Autodesk Inventor part; units mm, degrees
(part 2 of 2)
  spline S30 degree 3 poles (-13.3433, 65.0371) (-13.2374, 65.0737) (-13.0255, 65.1467) (-12.7024, 65.2399) (-12.4302, 65.3065) (-12.2106, 65.3513) (-12.0451, 65.3806) (-11.8787, 65.4045) (-11.6563, 65.4323) (-11.4592, 65.431) (-11.2933, 65.4596) (-11.2263, 65.4806) (-11.175, 65.5032) (-11.1385, 65.5242) (-11.1036, 65.5476) (-11.0712, 65.5745) (-11.0418, 65.6046) (-11.0157, 65.6376) (-10.9923, 65.6726) (-10.9749, 65.7109) (-10.9587, 65.7498) (-10.9463, 65.8046) (-10.9343, 65.8736) (-10.92, 65.9421) (-10.9113, 65.9976) (-10.912, 66.0397) (-10.914, 66.0817) (-10.9229, 66.1229) (-10.9349, 66.1632) (-10.9512, 66.202) (-10.9713, 66.239) (-10.9951, 66.2736) (-11.0213, 66.3066) (-11.0607, 66.3465) (-11.1152, 66.3908) (-11.2588, 66.4786) (-11.4424, 66.5501) (-11.6389, 66.658) (-11.7847, 66.7417) (-11.9277, 66.83) (-12.1153, 66.9527) (-12.3437, 67.115) (-12.6096, 67.3209) (-12.7795, 67.467) (-12.8645, 67.5401) knots 0 0 0 0 0.033613 0.067227 0.100839 0.117647 0.134454 0.151261 0.168068 0.201677 0.210077 0.218473 0.222676 0.226878 0.231076 0.235279 0.239479 0.24368 0.247882 0.252083 0.256283 0.260485 0.268889 0.277292 0.281494 0.285694 0.289895 0.294097 0.298298 0.302498 0.306701 0.310899 0.315101 0.319304 0.3277 0.3361 0.369709 0.386516 0.403323 0.420131 0.436938 0.470551 0.504164 0.537777 0.537777 0.537777 0.537777 projected
  arc A30 (-13.3433, 65.0371) -> (-13.4236, 64.2845) centre (6.5, 62.5385) ccw projected
  spline S31 degree 3 poles (-13.4839, 61.7369) (-13.3855, 61.7904) (-13.1885, 61.8974) (-12.8852, 62.0425) (-12.6276, 62.1529) (-12.4184, 62.2332) (-12.26, 62.2894) (-12.0998, 62.3404) (-11.885, 62.4044) (-11.6904, 62.4355) (-11.5315, 62.4911) (-11.4688, 62.5229) (-11.4219, 62.5536) (-11.3894, 62.5803) (-11.3588, 62.6091) (-11.3313, 62.641) (-11.3072, 62.6755) (-11.2869, 62.7123) (-11.2696, 62.7507) (-11.2587, 62.7914) (-11.2491, 62.8324) (-11.246, 62.8885) (-11.2455, 62.9585) (-11.2427, 63.0284) (-11.2432, 63.0846) (-11.2508, 63.126) (-11.2597, 63.1671) (-11.2752, 63.2063) (-11.2937, 63.2441) (-11.3162, 63.2797) (-11.3421, 63.3128) (-11.3713, 63.3431) (-11.4025, 63.3713) (-11.448, 63.4042) (-11.509, 63.4389) (-11.6652, 63.5019) (-11.858, 63.5422) (-12.0696, 63.6163) (-12.2272, 63.6748) (-12.3828, 63.7384) (-12.588, 63.8285) (-12.84, 63.951) (-13.1361, 64.1103) (-13.3278, 64.2265) (-13.4236, 64.2845) knots 0 0 0 0 0.033613 0.067227 0.100839 0.117647 0.134454 0.151261 0.168068 0.201677 0.210077 0.218473 0.222676 0.226878 0.231076 0.235279 0.239479 0.24368 0.247882 0.252083 0.256283 0.260485 0.268889 0.277292 0.281494 0.285694 0.289895 0.294097 0.298298 0.302498 0.306701 0.310899 0.315101 0.319304 0.3277 0.3361 0.369709 0.386516 0.403323 0.420131 0.436938 0.470551 0.504164 0.537777 0.537777 0.537777 0.537777 projected
  arc A31 (-13.4839, 61.7369) -> (-13.4393, 60.9814) centre (6.5, 62.5385) ccw projected
  spline S32 degree 3 poles (-13.0795, 58.4586) (-12.9911, 58.5276) (-12.8145, 58.6655) (-12.5391, 58.8586) (-12.3033, 59.0099) (-12.1101, 59.1235) (-11.9631, 59.205) (-11.8135, 59.2817) (-11.6121, 59.3802) (-11.4254, 59.4429) (-11.2777, 59.5238) (-11.2212, 59.5655) (-11.1799, 59.6035) (-11.1523, 59.6352) (-11.1268, 59.6687) (-11.105, 59.7046) (-11.0869, 59.7426) (-11.0729, 59.7823) (-11.0621, 59.8231) (-11.0581, 59.865) (-11.0554, 59.907) (-11.0616, 59.9628) (-11.0726, 60.0319) (-11.0813, 60.1014) (-11.0911, 60.1567) (-11.1054, 60.1963) (-11.121, 60.2354) (-11.1427, 60.2715) (-11.1672, 60.3057) (-11.1952, 60.3371) (-11.2262, 60.3655) (-11.26, 60.3906) (-11.2954, 60.4133) (-11.3457, 60.4382) (-11.4116, 60.4624) (-11.576, 60.4989) (-11.7728, 60.5068) (-11.9937, 60.5451) (-12.1588, 60.5769) (-12.3227, 60.614) (-12.54, 60.6692) (-12.8087, 60.7485) (-13.127, 60.8569) (-13.3352, 60.9399) (-13.4393, 60.9814) knots 0 0 0 0 0.033613 0.067227 0.100839 0.117647 0.134454 0.151261 0.168068 0.201677 0.210077 0.218473 0.222676 0.226878 0.231076 0.235279 0.239479 0.24368 0.247882 0.252083 0.256283 0.260485 0.268889 0.277292 0.281494 0.285694 0.289895 0.294097 0.298298 0.302498 0.306701 0.310899 0.315101 0.319304 0.3277 0.3361 0.369709 0.386516 0.403323 0.420131 0.436938 0.470551 0.504164 0.537777 0.537777 0.537777 0.537777 projected
  arc A32 (-13.0795, 58.4586) -> (-12.9111, 57.7207) centre (6.5, 62.5385) ccw projected
  spline S33 degree 3 poles (-12.1409, 55.2916) (-12.0651, 55.3741) (-11.9136, 55.5393) (-11.6738, 55.775) (-11.466, 55.9631) (-11.2942, 56.107) (-11.1626, 56.2116) (-11.0277, 56.3118) (-10.8453, 56.4421) (-10.6714, 56.5347) (-10.5391, 56.6388) (-10.4902, 56.6892) (-10.4557, 56.7335) (-10.4337, 56.7693) (-10.4141, 56.8065) (-10.3984, 56.8456) (-10.3869, 56.8861) (-10.3796, 56.9275) (-10.3757, 56.9695) (-10.3786, 57.0114) (-10.3829, 57.0533) (-10.3981, 57.1074) (-10.4204, 57.1738) (-10.4404, 57.2408) (-10.4591, 57.2938) (-10.4798, 57.3305) (-10.5016, 57.3665) (-10.529, 57.3985) (-10.5587, 57.4282) (-10.5915, 57.4546) (-10.6268, 57.4775) (-10.6643, 57.4967) (-10.7029, 57.5132) (-10.7566, 57.5296) (-10.8256, 57.5426) (-10.9937, 57.5515) (-11.1892, 57.5269) (-11.4134, 57.5283) (-11.5814, 57.5325) (-11.7493, 57.5422) (-11.9726, 57.5608) (-12.2507, 57.5948) (-12.5826, 57.6493) (-12.8016, 57.6969) (-12.9111, 57.7207) knots 0 0 0 0 0.033613 0.067227 0.100839 0.117647 0.134454 0.151261 0.168068 0.201677 0.210077 0.218473 0.222676 0.226878 0.231076 0.235279 0.239479 0.24368 0.247882 0.252083 0.256283 0.260485 0.268889 0.277292 0.281494 0.285694 0.289895 0.294097 0.298298 0.302498 0.306701 0.310899 0.315101 0.319304 0.3277 0.3361 0.369709 0.386516 0.403323 0.420131 0.436938 0.470551 0.504164 0.537777 0.537777 0.537777 0.537777 projected
  arc A33 (-12.1409, 55.2916) -> (-11.8534, 54.5915) centre (6.5, 62.5385) ccw projected
  spline S34 degree 3 poles (-10.6939, 52.3222) (-10.6327, 52.4161) (-10.5104, 52.6039) (-10.3127, 52.8759) (-10.1387, 53.0956) (-9.993, 53.2658) (-9.8804, 53.3907) (-9.7638, 53.5117) (-9.6053, 53.6703) (-9.449, 53.7903) (-9.3356, 53.9148) (-9.2957, 53.9725) (-9.269, 54.0219) (-9.2531, 54.0608) (-9.2399, 54.1007) (-9.2309, 54.1418) (-9.2262, 54.1837) (-9.2259, 54.2257) (-9.2289, 54.2678) (-9.2387, 54.3087) (-9.2498, 54.3493) (-9.2737, 54.4001) (-9.3066, 54.4619) (-9.3374, 54.5248) (-9.3646, 54.5739) (-9.391, 54.6067) (-9.4184, 54.6387) (-9.4507, 54.6657) (-9.485, 54.6901) (-9.5216, 54.7108) (-9.5602, 54.7276) (-9.6003, 54.7403) (-9.6412, 54.7502) (-9.6968, 54.7575) (-9.767, 54.759) (-9.9343, 54.7401) (-10.1231, 54.6837) (-10.3445, 54.6482) (-10.5109, 54.6247) (-10.678, 54.6066) (-10.9014, 54.5882) (-11.1813, 54.5759) (-11.5176, 54.5751) (-11.7414, 54.586) (-11.8534, 54.5915) knots 0 0 0 0 0.033613 0.067227 0.100839 0.117647 0.134454 0.151261 0.168068 0.201677 0.210077 0.218473 0.222676 0.226878 0.231076 0.235279 0.239479 0.24368 0.247882 0.252083 0.256283 0.260485 0.268889 0.277292 0.281494 0.285694 0.289895 0.294097 0.298298 0.302498 0.306701 0.310899 0.315101 0.319304 0.3277 0.3361 0.369709 0.386516 0.403323 0.420131 0.436938 0.470551 0.504164 0.537777 0.537777 0.537777 0.537777 projected
  arc A34 (-10.6939, 52.3222) -> (-10.295, 51.679) centre (6.5, 62.5385) ccw projected
  spline S35 degree 3 poles (-8.7778, 49.6316) (-8.733, 49.7342) (-8.6432, 49.9396) (-8.493, 50.2405) (-8.3576, 50.4858) (-8.2418, 50.6777) (-8.1513, 50.8193) (-8.0562, 50.9579) (-7.926, 51.1404) (-7.7915, 51.2844) (-7.7003, 51.4259) (-7.6703, 51.4895) (-7.6522, 51.5425) (-7.6429, 51.5836) (-7.6365, 51.6251) (-7.6343, 51.6671) (-7.6366, 51.7092) (-7.6432, 51.7507) (-7.6531, 51.7917) (-7.6695, 51.8304) (-7.6871, 51.8687) (-7.7191, 51.9149) (-7.7617, 51.9704) (-7.8024, 52.0273) (-7.8373, 52.0714) (-7.8687, 52.0993) (-7.901, 52.1263) (-7.9374, 52.1477) (-7.9752, 52.1661) (-8.0147, 52.1805) (-8.0556, 52.1907) (-8.0972, 52.1966) (-8.1391, 52.1997) (-8.1952, 52.1978) (-8.2647, 52.1876) (-8.4266, 52.1415) (-8.6035, 52.0548) (-8.816, 51.9833) (-8.9763, 51.9327) (-9.1382, 51.8873) (-9.3555, 51.8324) (-9.6296, 51.7743) (-9.9611, 51.7181) (-10.1837, 51.692) (-10.295, 51.679) knots 0 0 0 0 0.033613 0.067227 0.100839 0.117647 0.134454 0.151261 0.168068 0.201677 0.210077 0.218473 0.222676 0.226878 0.231076 0.235279 0.239479 0.24368 0.247882 0.252083 0.256283 0.260485 0.268889 0.277292 0.281494 0.285694 0.289895 0.294097 0.298298 0.302498 0.306701 0.310899 0.315101 0.319304 0.3277 0.3361 0.369709 0.386516 0.403323 0.420131 0.436938 0.470551 0.504164 0.537777 0.537777 0.537777 0.537777 projected
  arc A35 (-8.7778, 49.6316) -> (-8.2785, 49.0628) centre (6.5, 62.5385) ccw projected
  spline S36 degree 3 poles (-6.445, 47.2929) (-6.4177, 47.4016) (-6.363, 47.619) (-6.2643, 47.9404) (-6.1711, 48.2047) (-6.0885, 48.413) (-6.0226, 48.5676) (-5.9516, 48.72) (-5.8532, 48.9214) (-5.7443, 49.0856) (-5.6775, 49.2402) (-5.6585, 49.3078) (-5.6493, 49.3631) (-5.6469, 49.4051) (-5.6474, 49.4472) (-5.6522, 49.489) (-5.6613, 49.5301) (-5.6747, 49.5699) (-5.6912, 49.6087) (-5.7137, 49.6443) (-5.7374, 49.6791) (-5.7765, 49.7194) (-5.8277, 49.7671) (-5.8772, 49.8166) (-5.9189, 49.8543) (-5.9545, 49.8767) (-5.9908, 49.898) (-6.0302, 49.9131) (-6.0705, 49.9251) (-6.1119, 49.9327) (-6.1539, 49.9361) (-6.1959, 49.935) (-6.2378, 49.9312) (-6.2927, 49.92) (-6.3596, 49.8986) (-6.5117, 49.8264) (-6.672, 49.7118) (-6.8698, 49.6063) (-7.0196, 49.53) (-7.1718, 49.4586) (-7.3771, 49.3687) (-7.6379, 49.2663) (-7.9556, 49.1563) (-8.1709, 49.0939) (-8.2785, 49.0628) knots 0 0 0 0 0.033613 0.067227 0.100839 0.117647 0.134454 0.151261 0.168068 0.201677 0.210077 0.218473 0.222676 0.226878 0.231076 0.235279 0.239479 0.24368 0.247882 0.252083 0.256283 0.260485 0.268889 0.277292 0.281494 0.285694 0.289895 0.294097 0.298298 0.302498 0.306701 0.310899 0.315101 0.319304 0.3277 0.3361 0.369709 0.386516 0.403323 0.420131 0.436938 0.470551 0.504164 0.537777 0.537777 0.537777 0.537777 projected
  arc A36 (-6.445, 47.2929) -> (-5.859, 46.8141) centre (6.5, 62.5385) ccw projected
  spline S37 degree 3 poles (-3.7592, 45.3702) (-3.7501, 45.4819) (-3.7319, 45.7053) (-3.6875, 46.0386) (-3.639, 46.3146) (-3.5919, 46.5337) (-3.5522, 46.697) (-3.5073, 46.859) (-3.4434, 47.0739) (-3.363, 47.2538) (-3.3226, 47.4172) (-3.3149, 47.487) (-3.315, 47.5431) (-3.3196, 47.5849) (-3.3269, 47.6263) (-3.3386, 47.6668) (-3.3543, 47.7058) (-3.3741, 47.7429) (-3.3967, 47.7785) (-3.4248, 47.8098) (-3.4539, 47.8402) (-3.4992, 47.8736) (-3.5575, 47.9122) (-3.6145, 47.9529) (-3.6618, 47.9832) (-3.7006, 47.9994) (-3.7399, 48.0145) (-3.7812, 48.0229) (-3.823, 48.0281) (-3.8651, 48.0288) (-3.907, 48.0252) (-3.9483, 48.0173) (-3.989, 48.0066) (-4.0413, 47.9865) (-4.1038, 47.9544) (-4.242, 47.8581) (-4.3812, 47.7187) (-4.5589, 47.5821) (-4.6941, 47.4822) (-4.8324, 47.3867) (-5.0201, 47.2643) (-5.2605, 47.1203) (-5.5558, 46.9595) (-5.7579, 46.8625) (-5.859, 46.8141) knots 0 0 0 0 0.033613 0.067227 0.100839 0.117647 0.134454 0.151261 0.168068 0.201677 0.210077 0.218473 0.222676 0.226878 0.231076 0.235279 0.239479 0.24368 0.247882 0.252083 0.256283 0.260485 0.268889 0.277292 0.281494 0.285694 0.289895 0.294097 0.298298 0.302498 0.306701 0.310899 0.315101 0.319304 0.3277 0.3361 0.369709 0.386516 0.403323 0.420131 0.436938 0.470551 0.504164 0.537777 0.537777 0.537777 0.537777 projected
  arc A37 (-3.7592, 45.3702) -> (-3.1023, 44.9943) centre (6.5, 62.5385) ccw projected
  circle A38 centre (6.5, 62.5385) radius 16 projected
  circle A39 centre (16.1803, 34.1432) radius 4.0005 projected
  arc A40 (25.4036, 41.8198) -> (23.2102, 40.8992) centre (27.6407, 33.4167) ccw projected
  arc A41 (23.2102, 40.8992) -> (22.7103, 41.3835) centre (16.1803, 34.1432) ccw projected
  arc A42 (22.7103, 41.3835) -> (23.561, 43.6049) centre (15.0912, 45.5749) ccw projected
  arc A43 (23.561, 43.6049) -> (22.8672, 44.1074) centre (16.1803, 34.1432) ccw projected
  arc A44 (22.8672, 44.1074) -> (21.022, 42.606) centre (27.3812, 36.6749) ccw projected
  arc A45 (21.022, 42.606) -> (20.406, 42.9299) centre (16.1803, 34.1432) ccw projected
  arc A46 (20.406, 42.9299) -> (20.5964, 45.3011) centre (11.9147, 44.805) ccw projected
  arc A47 (20.5964, 45.3011) -> (19.7891, 45.5877) centre (16.1803, 34.1432) ccw projected
  arc A48 (19.7891, 45.5877) -> (18.4416, 43.6273) centre (26.2142, 39.728) ccw projected
  arc A49 (18.4416, 43.6273) -> (17.7593, 43.7645) centre (16.1803, 34.1432) ccw projected
  arc A50 (17.7593, 43.7645) -> (17.2739, 46.0932) centre (9.0837, 43.1713) ccw projected
  arc A51 (17.2739, 46.0932) -> (16.4186, 46.1408) centre (16.1803, 34.1432) ccw projected
  arc A52 (16.4186, 46.1408) -> (15.678, 43.8802) centre (24.2344, 42.3286) ccw projected
  arc A53 (15.678, 43.8802) -> (14.9847, 43.8196) centre (16.1803, 34.1432) ccw projected
  arc A54 (14.9847, 43.8196) -> (13.8629, 45.9173) centre (6.8276, 40.8063) ccw projected
  arc A55 (13.8629, 45.9173) -> (13.0289, 45.722) centre (16.1803, 34.1432) ccw projected
  arc A56 (13.0289, 45.722) -> (12.9551, 43.3443) centre (21.602, 44.2662) ccw projected
  arc A57 (12.9551, 43.3443) -> (12.307, 43.0908) centre (16.1803, 34.1432) ccw projected
  arc A58 (12.307, 43.0908) -> (10.6396, 44.7875) centre (5.3292, 37.9014) ccw projected
  arc A59 (10.6396, 44.7875) -> (9.8944, 44.3651) centre (16.1803, 34.1432) ccw projected
  arc A60 (9.8944, 44.3651) -> (10.4935, 42.063) centre (18.5304, 45.3836) ccw projected
  arc A61 (10.4935, 42.063) -> (9.943, 41.6371) centre (16.1803, 34.1432) ccw projected
  arc A62 (9.943, 41.6371) -> (7.8652, 42.7953) centre (4.71, 34.6921) ccw projected
  arc A63 (7.8652, 42.7953) -> (7.2692, 42.1801) centre (16.1803, 34.1432) ccw projected
  arc A64 (7.2692, 42.1801) -> (8.4926, 40.14) centre (15.2684, 45.5904) ccw projected
  arc A65 (8.4926, 40.14) -> (8.0844, 39.5763) centre (16.1803, 34.1432) ccw projected
  arc A66 (8.0844, 39.5763) -> (5.7645, 40.1022) centre (5.0199, 31.4383) ccw projected
  arc A67 (5.7645, 40.1022) -> (5.3659, 39.344) centre (16.1803, 34.1432) ccw projected
  arc A68 (5.3659, 39.344) -> (7.1145, 37.7312) centre (12.0803, 44.8698) ccw projected
  arc A69 (7.1145, 37.7312) -> (6.8816, 37.0753) centre (16.1803, 34.1432) ccw projected
  arc A70 (6.8816, 37.0753) -> (4.5075, 36.9264) centre (6.2341, 28.4036) ccw projected
  arc A71 (4.5075, 36.9264) -> (4.3387, 36.0865) centre (16.1803, 34.1432) ccw projected
  arc A72 (4.3387, 36.0865) -> (6.4709, 35.0318) centre (9.2244, 43.2802) ccw projected
  arc A73 (6.4709, 35.0318) -> (6.4322, 34.3368) centre (16.1803, 34.1432) ccw projected
  arc A74 (6.4322, 34.3368) -> (4.1962, 33.525) centre (8.254, 25.8339) ccw projected
  arc A75 (4.1962, 33.525) -> (4.2709, 32.6717) centre (16.1803, 34.1432) ccw projected
  arc A76 (4.2709, 32.6717) -> (6.6138, 32.2603) centre (6.9319, 40.9503) ccw projected
  arc A77 (6.6138, 32.2603) -> (6.7725, 31.5826) centre (16.1803, 34.1432) ccw projected
  arc A78 (6.7725, 31.5826) -> (4.8558, 30.1738) centre (10.916, 23.9374) ccw projected
  arc A79 (4.8558, 30.1738) -> (5.1679, 29.376) centre (16.1803, 34.1432) ccw projected
  arc A80 (5.1679, 29.376) -> (7.5318, 29.6414) centre (5.3888, 38.069) ccw projected
  arc A81 (7.5318, 29.6414) -> (7.875, 29.0359) centre (16.1803, 34.1432) ccw projected
  arc A82 (7.875, 29.0359) -> (6.4329, 27.1441) centre (14.0046, 22.8677) ccw projected
  arc A83 (6.4329, 27.1441) -> (6.957, 26.4665) centre (16.1803, 34.1432) ccw projected
  arc A84 (6.957, 26.4665) -> (9.1504, 27.3872) centre (4.7198, 34.8697) ccw projected
  arc A85 (9.1504, 27.3872) -> (9.6503, 26.9029) centre (16.1803, 34.1432) ccw projected
  arc A86 (9.6503, 26.9029) -> (8.7996, 24.6814) centre (17.2694, 22.7115) ccw projected
  arc A87 (8.7996, 24.6814) -> (9.4934, 24.179) centre (16.1803, 34.1432) ccw projected
  arc A88 (9.4934, 24.179) -> (11.3386, 25.6803) centre (4.9794, 31.6115) ccw projected
  arc A89 (11.3386, 25.6803) -> (11.9546, 25.3565) centre (16.1803, 34.1432) ccw projected
  arc A90 (11.9546, 25.3565) -> (11.7642, 22.9853) centre (20.4459, 23.4814) ccw projected
  arc A91 (11.7642, 22.9853) -> (12.5715, 22.6987) centre (16.1803, 34.1432) ccw projected
  arc A92 (12.5715, 22.6987) -> (13.919, 24.659) centre (6.1464, 28.5584) ccw projected
  arc A93 (13.919, 24.659) -> (14.6013, 24.5219) centre (16.1803, 34.1432) ccw projected
  arc A94 (14.6013, 24.5219) -> (15.0867, 22.1931) centre (23.2769, 25.115) ccw projected
  arc A95 (15.0867, 22.1931) -> (15.9419, 22.1455) centre (16.1803, 34.1432) ccw projected
  arc A96 (15.9419, 22.1455) -> (16.6826, 24.4061) centre (8.1262, 25.9577) ccw projected
  arc A97 (16.6826, 24.4061) -> (17.3759, 24.4668) centre (16.1803, 34.1432) ccw projected
  arc A98 (17.3759, 24.4668) -> (18.4977, 22.3691) centre (25.533, 27.4801) ccw projected
  arc A99 (18.4977, 22.3691) -> (19.3317, 22.5644) centre (16.1803, 34.1432) ccw projected
  arc A100 (19.3317, 22.5644) -> (19.4055, 24.942) centre (10.7586, 24.0202) ccw projected
  arc A101 (19.4055, 24.942) -> (20.0536, 25.1956) centre (16.1803, 34.1432) ccw projected
  arc A102 (20.0536, 25.1956) -> (21.721, 23.4989) centre (27.0313, 30.3849) ccw projected
  arc A103 (21.721, 23.4989) -> (22.4662, 23.9213) centre (16.1803, 34.1432) ccw projected
  arc A104 (22.4662, 23.9213) -> (21.8671, 26.2234) centre (13.8302, 22.9028) ccw projected
  arc A105 (21.8671, 26.2234) -> (22.4176, 26.6493) centre (16.1803, 34.1432) ccw projected
  arc A106 (22.4176, 26.6493) -> (24.4954, 25.491) centre (27.6506, 33.5943) ccw projected
  arc A107 (24.4954, 25.491) -> (25.0914, 26.1063) centre (16.1803, 34.1432) ccw projected
  arc A108 (25.0914, 26.1063) -> (23.868, 28.1463) centre (17.0922, 22.696) ccw projected
  arc A109 (23.868, 28.1463) -> (24.2762, 28.7101) centre (16.1803, 34.1432) ccw projected
  arc A110 (24.2762, 28.7101) -> (26.5961, 28.1841) centre (27.3406, 36.8481) ccw projected
  arc A111 (26.5961, 28.1841) -> (26.9947, 28.9424) centre (16.1803, 34.1432) ccw projected
  arc A112 (26.9947, 28.9424) -> (25.2461, 30.5551) centre (20.2803, 23.4166) ccw projected
  arc A113 (25.2461, 30.5551) -> (25.4789, 31.211) centre (16.1803, 34.1432) ccw projected
  arc A114 (25.4789, 31.211) -> (27.8531, 31.36) centre (26.1265, 39.8827) ccw projected
  arc A115 (27.8531, 31.36) -> (28.0219, 32.1998) centre (16.1803, 34.1432) ccw projected
  arc A116 (28.0219, 32.1998) -> (25.8897, 33.2546) centre (23.1362, 25.0062) ccw projected
  arc A117 (25.8897, 33.2546) -> (25.9284, 33.9495) centre (16.1803, 34.1432) ccw projected
  arc A118 (25.9284, 33.9495) -> (28.1644, 34.7613) centre (24.1066, 42.4524) ccw projected
  arc A119 (28.1644, 34.7613) -> (28.0897, 35.6147) centre (16.1803, 34.1432) ccw projected
  arc A120 (28.0897, 35.6147) -> (25.7468, 36.026) centre (25.4287, 27.336) ccw projected
  arc A121 (25.7468, 36.026) -> (25.5881, 36.7037) centre (16.1803, 34.1432) ccw projected
  arc A122 (25.5881, 36.7037) -> (27.5048, 38.1126) centre (21.4446, 44.3489) ccw projected
  arc A123 (27.5048, 38.1126) -> (27.1927, 38.9104) centre (16.1803, 34.1432) ccw projected
  arc A124 (27.1927, 38.9104) -> (24.8288, 38.645) centre (26.9718, 30.2173) ccw projected
  arc A125 (24.8288, 38.645) -> (24.4856, 39.2505) centre (16.1803, 34.1432) ccw projected
  arc A126 (24.4856, 39.2505) -> (25.9277, 41.1423) centre (18.356, 45.4186) ccw projected
  arc A127 (25.9277, 41.1423) -> (25.4036, 41.8198) centre (16.1803, 34.1432) ccw projected
  arc A128 (11.7246, 16.8961) -> (10.2227, 15.407) centre (14.2615, 12.8353) ccw projected
  arc A129 (10.2227, 15.407) -> (10.7174, 14.6349) centre (15.375, 18.1635) ccw projected
  arc A130 (10.7174, 14.6349) -> (12.6979, 15.377) centre (10.0692, 19.3789) ccw projected
  arc A131 (12.6979, 15.377) -> (13.1667, 14.9925) centre (15.375, 18.1635) ccw projected
  arc A132 (13.1667, 14.9925) -> (12.8269, 12.905) centre (17.606, 13.1984) ccw projected
  arc A133 (12.8269, 12.905) -> (13.6809, 12.5712) centre (15.375, 18.1635) ccw projected
  arc A134 (13.6809, 12.5712) -> (14.847, 14.3356) centre (10.3681, 16.0281) ccw projected
  arc A135 (14.847, 14.3356) -> (15.4523, 14.3001) centre (15.375, 18.1635) ccw projected
  arc A136 (15.4523, 14.3001) -> (16.4044, 12.4116) centre (20.0983, 15.458) ccw projected
  arc A137 (16.4044, 12.4116) -> (17.2915, 12.6434) centre (15.375, 18.1635) ccw projected
  arc A138 (17.2915, 12.6434) -> (17.1978, 14.7563) centre (12.5794, 13.493) ccw projected
  arc A139 (17.1978, 14.7563) -> (17.7084, 15.0834) centre (15.375, 18.1635) ccw projected
  arc A140 (17.7084, 15.0834) -> (19.5887, 14.1152) centre (20.7864, 18.751) ccw projected
  arc A141 (19.5887, 14.1152) -> (20.1701, 14.8242) centre (15.375, 18.1635) ccw projected
  arc A142 (20.1701, 14.8242) -> (18.8524, 16.4784) centre (15.8586, 12.7418) ccw projected
  arc A143 (18.8524, 16.4784) -> (19.0731, 17.0432) centre (15.375, 18.1635) ccw projected
  arc A144 (19.0731, 17.0432) -> (21.1635, 17.365) centre (19.4076, 21.8195) ccw projected
  arc A145 (21.1635, 17.365) -> (21.2171, 18.2804) centre (15.375, 18.1635) ccw projected
  arc A146 (21.2171, 18.2804) -> (19.1787, 18.8442) centre (18.953, 14.0615) ccw projected
  arc A147 (19.1787, 18.8442) -> (19.0254, 19.4308) centre (15.375, 18.1635) ccw projected
  arc A148 (19.0254, 19.4308) -> (20.5273, 20.9199) centre (16.4885, 23.4916) ccw projected
  arc A149 (20.5273, 20.9199) -> (20.0326, 21.692) centre (15.375, 18.1635) ccw projected
  arc A150 (20.0326, 21.692) -> (18.0521, 20.9499) centre (20.6808, 16.948) ccw projected
  arc A151 (18.0521, 20.9499) -> (17.5833, 21.3344) centre (15.375, 18.1635) ccw projected
  arc A152 (17.5833, 21.3344) -> (17.9231, 23.4219) centre (13.144, 23.1285) ccw projected
  arc A153 (17.9231, 23.4219) -> (17.0691, 23.7558) centre (15.375, 18.1635) ccw projected
  arc A154 (17.0691, 23.7558) -> (15.903, 21.9913) centre (20.3819, 20.2988) ccw projected
  arc A155 (15.903, 21.9913) -> (15.2977, 22.0268) centre (15.375, 18.1635) ccw projected
  arc A156 (15.2977, 22.0268) -> (14.3456, 23.9153) centre (10.6517, 20.8689) ccw projected
  arc A157 (14.3456, 23.9153) -> (13.4585, 23.6835) centre (15.375, 18.1635) ccw projected
  arc A158 (13.4585, 23.6835) -> (13.5522, 21.5706) centre (18.1706, 22.8339) ccw projected
  arc A159 (13.5522, 21.5706) -> (13.0416, 21.2435) centre (15.375, 18.1635) ccw projected
  arc A160 (13.0416, 21.2435) -> (11.1613, 22.2118) centre (9.9636, 17.5759) ccw projected
  arc A161 (11.1613, 22.2118) -> (10.5799, 21.5027) centre (15.375, 18.1635) ccw projected
  arc A162 (10.5799, 21.5027) -> (11.8976, 19.8485) centre (14.8914, 23.5851) ccw projected
  arc A163 (11.8976, 19.8485) -> (11.6769, 19.2837) centre (15.375, 18.1635) ccw projected
  arc A164 (11.6769, 19.2837) -> (9.5865, 18.9619) centre (11.3424, 14.5074) ccw projected
  arc A165 (9.5865, 18.9619) -> (9.5329, 18.0465) centre (15.375, 18.1635) ccw projected
  arc A166 (9.5329, 18.0465) -> (11.5713, 17.4827) centre (11.797, 22.2654) ccw projected
  arc A167 (11.5713, 17.4827) -> (11.7246, 16.8961) centre (15.375, 18.1635) ccw projected
  circle A168 centre (23.5, 78.5385) radius 3.5
  circle A169 centre (5, 20) radius 3.5
  line L0 (29.5, 0) -> (29.5, 88.5385) projected
  line L1 (0, 88.5385) -> (29.5, 88.5385) projected
  circle A170 centre (23.5, 78.5385) radius 1.5
  line L2 (0, 88.5385) -> (0, 0) projected
  circle A171 centre (5, 20) radius 1.5
  line L3 (0, 0) -> (29.5, 0) projected
  point P0 (0, -0.9615)
  dimension "d7" = 7
  dimension "d11" = 7
  dimension "d12" = 6
  dimension "d13" = 10
  dimension "d14" = 3
  dimension "d15" = 5
  dimension "d16" = 3
  dimension "d17" = 20
  constraints: 4 centre point, 4 coincident
  measures "d7" diameter of A169
  measures "d11" diameter of A168
  measures "d12" distance from line of L0 A168.centre
  measures "d13" distance from line of L1 A168.centre
  measures "d14" diameter of A170
  measures "d15" distance from line of A169.centre L2
  measures "d16" diameter of A171
  measures "d17" distance from line of L3 A169.centre
hole "Hole1" at (-22.5, 79.5, 23.5) at (-22.5, 20.9615, 5) direction (1, 0, 0) diameter 3.6 end through all countersink diameter 6.7 countersink angle 90 clearance for "Countersunk Flat Head Screw ISO 2009/7046" size "M3" standard "ISO"
sketch "Sketch7" plane through (-22.5, 0.9615, 29.5) normal (0, 0, 1) x (1, 0, 0)
  line L0 (0, 11.7202) -> (0, 24.6067) projected
  line L1 (0, 56.8885) -> (0, 68.1885) projected
  line L2 (1.55, 80.3385) -> (1.55, 76.7385) projected
  line L3 (6, 24.6067) -> (6, 11.7202) projected
  line L4 (0, 11.7202) -> (6, 11.7202)
  line L5 (6, 11.7202) -> (6, 24.6067)
  line L6 (6, 24.6067) -> (0, 24.6067)
  line L7 (0, 24.6067) -> (0, 11.7202)
  line L8 (6, 0) -> (6, 88.5385) projected
  line L9 (0, 56.8885) -> (6, 56.8885)
  line L10 (6, 56.8885) -> (6, 68.1885)
  line L11 (6, 68.1885) -> (0, 68.1885)
  line L12 (0, 68.1885) -> (0, 56.8885)
  line L13 (0, 88.5385) -> (0, 0) projected
  line L14 (6, 80.3385) -> (1.55, 80.3385) projected
  line L15 (0, 76.7385) -> (6, 76.7385)
  line L16 (6, 76.7385) -> (6, 80.3385)
  line L17 (6, 80.3385) -> (0, 80.3385)
  line L18 (0, 80.3385) -> (0, 76.7385)
  line L19 (0, 11.7202) -> (6, 0)
  line L20 (6, 11.7202) -> (0, 0)
  line L21 (6, 24.6067) -> (0, 56.8885)
  line L22 (0, 24.6067) -> (6, 56.8885)
  line L23 (6, 68.1885) -> (0, 76.7385)
  line L24 (0, 68.1885) -> (6, 76.7385)
  point P0 (22.5, -0.9615)
  point P1 (3, 72.4635)
  point P2 (3, 40.7476)
  point P3 (3, 5.8601)
  constraints: 36 end point, 6 parallel, 5 point on line, 3 horizontal, 3 midpoint, 3 perpendicular, 2 other
hole "Hole2" at (-19.5, 73.425, 29.5) at (-19.5, 41.7091, 29.5) at (-19.5, 6.8216, 29.5) direction (0, 0, -1) diameter 3.6 end through all countersink diameter 6.6 countersink angle 90 clearance for "Countersunk Flat Head Screw ISO 2009/7046" size "M3" standard "ISO"
sketch "Sketch8" plane through (-22.5, 89.5, 0) normal (0, 1, 0) x (1, 0, 0)
  line L0 (0, -29.5) -> (6, -29.5) projected
  line L1 (6, 0) -> (6, -29.5) projected
  line L2 (6, 0) -> (0, 0) projected
  line L3 (0, 0) -> (0, -29.5) projected
  line L4 (0, 0) -> (0, -29.5) projected
  line L5 (0, -14.75) -> (6, -29.5)
  line L6 (6, -29.5) -> (6, -15.375)
  line L7 (6, -8.9317) -> (6, -21.8183) projected
  line L8 (0, 0) -> (6, 0) projected
  line L9 (6, -15.375) -> (0, 0)
  line L10 (0, 0) -> (0, -14.75)
  point P0 (22.5, 0)
  point P1 (3, -7.6875)
  point P2 (3, -22.125)
  constraints: 8 end point, 4 midpoint, 1 parallel
hole "Hole3" at (-19.5, 89.5, 7.6875) at (-19.5, 89.5, 22.125) direction (0, -1, 0) diameter 4 depth 3.75 counterbore diameter 4.6 counterbore depth 0.75
body "Solid1"
